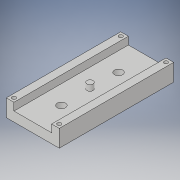
# Autodesk Inventor part: CameraLinearSupporter
Saved by Autodesk Inventor 2019 (Build 230136000, 136)
## iProperties
Created: 2019-08-08
Part Number: CameraLinearSupporter
Material: Generic
Document SubType Name: Modeling
Designer: aorfi
Density: 1 g/cm^3
Appearance: Default
Author: aorfi
Autodesk Inventor part; units mm, degrees
ref_plane "YZ Plane" through (0, 0, 0) normal (1, 0, 0) x (0, 1, 0)
ref_plane "XZ Plane" through (0, 0, 0) normal (0, 1, 0) x (-1, 0, 0)
ref_plane "XY Plane" through (0, 0, 0) normal (0, 0, 1) x (1, 0, 0)
sketch "Sketch1" plane through (0, 0, 0) normal (0, 1, 0) x (-1, 0, 0)
  line L0 (-13.8735, 30) -> (13.8735, 30)
  line L1 (13.8735, 30) -> (13.8735, -30)
  line L2 (13.8735, -30) -> (-13.8735, -30)
  line L3 (-13.8735, -30) -> (-13.8735, 30)
  line L4 (-13.8735, 30) -> (13.8735, -30) construction
  line L5 (13.8735, 30) -> (-13.8735, -30) construction
  point P0 (0, 0)
  dimension "d0" = 60
  dimension "d1" = 27.747
  constraints: 12 end point, 2 midpoint, 2 parallel, 1 horizontal, 1 perpendicular
  measures "d0" distance of L0.end L1.end
  measures "d1" distance of L1.end L2.end
extrude "Extrusion1" add sketch "Sketch1" along normal mid plane 5
sketch "Sketch2" plane through (0, 2.5, 0) normal (0, 1, 0) x (1, 0, 0)
  line L0 (-13.8735, -30) -> (13.8735, -30) projected
  line L1 (-13.8735, -30) -> (-9.8735, -30)
  line L2 (-9.8735, -30) -> (-9.8735, 30)
  line L3 (-9.8735, 30) -> (-13.8735, 30)
  line L4 (-13.8735, 30) -> (-13.8735, -30)
  line L5 (13.8735, 30) -> (-13.8735, 30) projected
  line L6 (13.8735, -30) -> (9.8735, -30)
  line L7 (9.8735, -30) -> (9.8735, 30)
  line L8 (9.8735, 30) -> (13.8735, 30)
  line L9 (13.8735, 30) -> (13.8735, -30)
  point P0 (0, 0)
  dimension "d4" = 4
  dimension "d5" = 4
  constraints: 16 end point, 4 parallel, 2 horizontal, 2 perpendicular, 1 collinear, 1 point on line
  measures "d4" distance between parallel lines of L4 L2
  measures "d5" distance between parallel lines of L9 L7
extrude "Extrusion2" add sketch "Sketch2" along normal blind 4 contours L4 L3 L2 L0 | L7 L5 L9 L0
sketch "Sketch3" plane through (0, 2.5, 0) normal (0, 1, 0) x (1, 0, 0)
  circle A0 centre (0, 0) radius 1.5875
  dimension "d8" = 3.175
  constraints: 1 centre point, 1 coincident
  measures "d8" diameter of A0
extrude "Extrusion3" add sketch "Sketch3" along normal blind 3
sketch "Sketch4" plane through (0, 2.5, 0) normal (0, 1, 0) x (1, 0, 0)
  line L0 (0, 0) -> (0, -30) construction
  line L1 (0, 0) -> (0, 30) construction
  line L2 (-9.8735, -30) -> (9.8735, -30) construction
  line L3 (9.8735, 30) -> (-9.8735, 30) construction
  point P0 (0, -15)
  point P1 (0, 15)
  constraints: 4 end point, 4 midpoint, 2 vertical
hole "Hole1" at (0, 2.5, 15) at (0, 2.5, -15) direction (0, -1, 0) diameter 4.305 end through all clearance for "Flat Head Machine Screw (82)" size "#6" standard "Ansi Unified Screw Threads"
sketch "Sketch5" plane through (0, 6.5, 0) normal (0, 1, 0) x (1, 0, 0)
  circle A0 centre (-11.8735, 28) radius 1
  circle A1 centre (-11.8735, -28) radius 1
  circle A2 centre (11.8735, -28) radius 1
  circle A3 centre (11.8735, 28) radius 1
  line L0 (-9.8735, 30) -> (-13.8735, 30) projected
  line L1 (13.8735, 30) -> (9.8735, 30) projected
  line L2 (-13.8735, -30) -> (-9.8735, -30) projected
  point P0 (0, 0)
  point P1 (-11.8735, 30)
  point P2 (11.8735, 30)
  dimension "d18" = 2
  dimension "d19" = 2
  dimension "d20" = 2
  constraints: 4 centre point, 4 vertical alignment, 3 equal radius, 2 horizontal alignment, 2 midpoint
  measures "d18" diameter of A0
  measures "d19" distance from line of L0 A0.centre
  measures "d20" distance from line of L2 A1.centre
extrude "Extrusion4" cut sketch "Sketch5" against normal blind 3
equation "\"d5\" = d4"
equation "\"d20\" = d19"
equation "\"BendRadius\" = Thickness"
equation "\"BendReliefWidth\" = Thickness"
equation "\"BendReliefDepth\" = 0.5 * Thickness"
equation "\"CornerReliefSize\" = 4 * Thickness"
equation "\"MinimumRemnant\" = 2 * Thickness"
equation "\"TransitionRadius\" = BendRadius"
equation "\"JacobiRadiusSize\" = Thickness"
equation "\"GapSize\" = Thickness"
equation "\"Thickness\" = 0.5"
body "Solid1"
